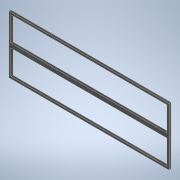
# Autodesk Inventor part: Grade
Saved by Autodesk Inventor 2022 (Build 260153000, 153)
## iProperties
Created: 2021-09-17
Part Number: Grade
Material: Genérico
Document SubType Name: Modeling
Designer: rubia
Density: 1 g/cm^3
Appearance: Cinza escuro
Author: rubia
Autodesk Inventor part; units mm, degrees
ref_plane "YZ Plane" through (0, 0, 0) normal (1, 0, 0) x (0, 1, 0)
ref_plane "XZ Plane" through (0, 0, 0) normal (0, 1, 0) x (-1, 0, 0)
ref_plane "XY Plane" through (0, 0, 0) normal (0, 0, 1) x (1, 0, 0)
sketch "Esboço1" plane through (0, 0, 0) normal (0, 0, 1) x (1, 0, 0)
  line L0 (0, 0) -> (150, 0)
  line L1 (150, 0) -> (150, 27)
  line L2 (150, 27) -> (0, 27)
  line L3 (0, 27) -> (0, 0)
  line L4 (2, 25) -> (148, 25)
  line L5 (148, 25) -> (148, 2)
  line L6 (148, 2) -> (2, 2)
  line L7 (2, 2) -> (2, 25)
  line L8 (0, 27) -> (150, 27) construction
  line L9 (0, 54) -> (150, 54)
  line L10 (150, 54) -> (150, 27)
  line L11 (0, 27) -> (0, 54)
  line L12 (2, 29) -> (148, 29)
  line L13 (148, 29) -> (148, 52)
  line L14 (148, 52) -> (2, 52)
  line L15 (2, 52) -> (2, 29)
  dimension "d6" = 150
  dimension "d7" = 27
  dimension "d8" = 2
  dimension "d9" = 2
  dimension "d10" = 2
  dimension "d11" = 2
  constraints: 32 end point, 6 symmetric about line, 5 parallel, 2 horizontal, 2 perpendicular
  measures "d6" distance of L2.end L1.end
  measures "d7" distance of L1.end L0.end
  measures "d8" distance between parallel lines of L2 L4
  measures "d9" distance between parallel lines of L0 L6
  measures "d10" distance between parallel lines of L3 L7
  measures "d11" distance between parallel lines of L1 L5
extrude "Extrusão1" add sketch "Esboço1" along normal blind 2
